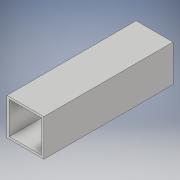
# Autodesk Inventor part: SUP_019_ClimberCrossBar
Saved by Autodesk Inventor 2018.3 (Build 223284000, 284)
## iProperties
Created: 2020-02-16
Part Number: SUP_019_ClimberCrossBar
Material: Generic
Document SubType Name: Modeling
Designer: 22turnmaxw
Density: 1 g/cm^3
Appearance: Default
Author: 22turnmaxw
Autodesk Inventor part; units mm, degrees
ref_plane "YZ Plane" through (0, 0, 0) normal (1, 0, 0) x (0, 1, 0)
ref_plane "XZ Plane" through (0, 0, 0) normal (0, 1, 0) x (-1, 0, 0)
ref_plane "XY Plane" through (0, 0, 0) normal (0, 0, 1) x (1, 0, 0)
sketch "Sketch1" plane through (0, 0, 0) normal (0, 0, 1) x (1, 0, 0)
  line L0 (0, 0) -> (25.4, 0)
  line L1 (25.4, 0) -> (25.4, 25.4)
  line L2 (25.4, 25.4) -> (0, 25.4)
  line L3 (0, 25.4) -> (0, 0)
  line L4 (1.5875, 23.8125) -> (23.8125, 23.8125)
  line L5 (23.8125, 23.8125) -> (23.8125, 1.5875)
  line L6 (23.8125, 1.5875) -> (1.5875, 1.5875)
  line L7 (1.5875, 1.5875) -> (1.5875, 23.8125)
  dimension "d0" = 25.4
  dimension "d1" = 25.4
  dimension "d2" = 1.5875
  constraints: 16 end point, 4 parallel, 2 perpendicular, 1 horizontal, 3 other
  measures "d0" distance of L1.end L2.end
  measures "d1" distance of L0.end L1.end
  measures "d2" distance between parallel lines of L4 L2
extrude "Extrusion1" add sketch "Sketch1" along normal blind 88.9
body "Solid1"
